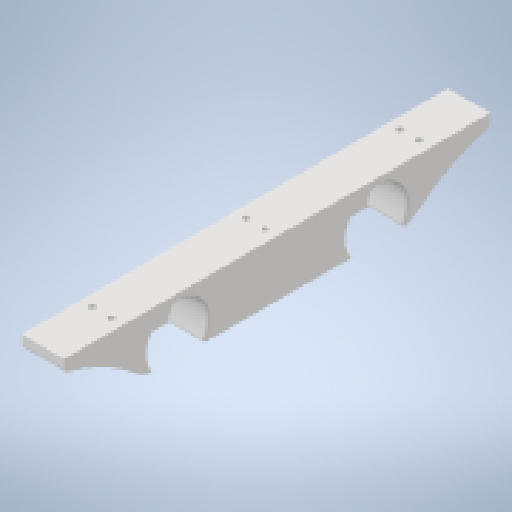
# Autodesk Inventor part: fasteners_motors
Saved by Autodesk Inventor 2023 (Build 270158000, 158)
## iProperties
Created: 2026-02-10
Part Number: fasteners_motors
Material: Типовые
Document SubType Name: Modeling
Designer: garin
Density: 1 g/cm^3
Appearance: По умолчанию
Author: garin
Autodesk Inventor part; units mm, degrees
ref_plane "YZ Plane" through (0, 0, 0) normal (1, 0, 0) x (0, 1, 0)
ref_plane "XY Plane" through (0, 0, 0) normal (0, 0, 1) x (1, 0, 0)
sketch "Эскиз1" plane through (0, 0, 0) normal (1, 0, 0) x (0, 1, 0)
  line L0 (0.0001, 0) -> (0.0001, -90)
  line L1 (0.0001, -90) -> (-4.9999, -90)
  line L2 (0.0001, -42) -> (0.0001, 0)
  circle A0 centre (-15.7559, -42) radius 12.6
  line L3 (-15.7559, -50.5) -> (-15.7559, -33.5) construction
  circle A1 centre (-15.7559, -50.5) radius 1.5
  circle A2 centre (-15.7559, -33.5) radius 1.5
  circle A3 centre (-15.7559, -42) radius 4
  line L4 (0.0001, 0) -> (-23.6599, 0)
  line L5 (-23.6599, 0) -> (-23.6599, -32.1874)
  line L6 (-23.6599, -32.1874) -> (-23.6599, -51.8126)
  arc A4 (-4.9999, -90) -> (-20.9999, -59) centre (-75.6064, -106.8131) ccw
  arc A5 (-23.6599, -51.8126) -> (-20.9999, -59) centre (-10.3066, -50.9566) ccw
  line L7 (40.5935, 0) -> (-48.1218, 0) construction
  line L8 (0.0001, 0) -> (0.0001, 90)
  line L9 (0.0001, 90) -> (-4.9999, 90)
  line L10 (0.0001, 42) -> (0.0001, 0)
  circle A6 centre (-15.7559, 42) radius 12.6
  line L11 (-15.7559, 50.5) -> (-15.7559, 33.5) construction
  circle A7 centre (-15.7559, 50.5) radius 1.5
  circle A8 centre (-15.7559, 33.5) radius 1.5
  circle A9 centre (-15.7559, 42) radius 4
  line L12 (-23.6599, 0) -> (-23.6599, 32.1874)
  line L13 (-23.6599, 32.1874) -> (-23.6599, 51.8126)
  arc A10 (-20.9999, 59) -> (-4.9999, 90) centre (-75.6064, 106.8131) ccw
  arc A11 (-20.9999, 59) -> (-23.6599, 51.8126) centre (-10.3066, 50.9566) ccw
  dimension "d34" = 90
  dimension "d35" = 5
  dimension "d38" = 25.2
  dimension "d39" = 8.5
  dimension "d40" = 17
  dimension "d41" = 3
  dimension "d42" = 3
  dimension "d43" = 8
  dimension "d44" = 23.66
  constraints: 28 end point, 14 symmetric about line, 12 centre point, 12 point on circle, 6 coincident, 3 perpendicular, 2 point on line, 1 horizontal, 1 vertical, 6 other
  measures "d34" distance of L0.start L0.end
  measures "d35" distance of L0.end L1.end
  measures "d38" diameter of A0
  measures "d39" distance of A0.centre L3.start
  measures "d40" distance of L3.start L3.end
  measures "d41" diameter of A1
  measures "d42" diameter of A2
  measures "d43" diameter of A3
  measures "d44" distance of L0.start L4.end
extrude "Выдавливание1" add sketch "Эскиз1" along normal blind 18 contours L0 L1 A4 A5 A0 L5 L4 | L4 L12 A6 A11 A10 L9 L8
extrude "Выдавливание2" add sketch "Эскиз1" along normal blind 3 contours A0 L6 | L13 A6 picked at (-22.3586, -42) picked at (-22.3586, 42)
chamfer "Фаска1" distance 2 angle 45 4 edges at (0, -17.2559, -33.5) (0, -17.2559, -50.5) (0, -17.2559, 50.5) (0, -17.2559, 33.5)
fillet "Сопряжение1" radius 1 6 edges at (10.5, -23.6599, -32.1874) (10.5, -23.6599, -51.8126) (18, -3.1559, -42) (18, -3.1559, 42) (10.5, -23.6599, 32.1874) (10.5, -23.6599, 51.8126)
fillet "Сопряжение2" radius 2 2 edges at (9, -4.9999, -90) (9, -4.9999, 90)
sketch "Эскиз2" plane through (0, 0.0001, 90) normal (0, 1, 0) x (1, 0, 0)
  line L0 (18, 180) -> (18, 0) projected
  line L1 (0, 0) -> (18, 0) projected
  line L2 (18, 180) -> (13, 180)
  line L3 (13, 180) -> (13, 0)
  line L4 (13, 0) -> (18, 0)
  line L5 (18, 0) -> (18, 180)
  line L6 (0, 180) -> (0, 0) projected
  line L7 (18, 0) -> (0, 0)
  line L8 (0, 0) -> (0, 25)
  line L9 (0, 25) -> (18, 25)
  line L10 (18, 25) -> (18, 0)
  line L11 (0, 180) -> (18, 180) projected
  line L12 (0, 0) -> (5, 0)
  line L13 (5, 0) -> (5, 180)
  line L14 (5, 180) -> (0, 180)
  line L15 (0, 180) -> (0, 0)
  line L16 (18, 180) -> (0, 180)
  line L17 (0, 180) -> (0, 155)
  line L18 (0, 155) -> (18, 155)
  line L19 (18, 155) -> (18, 180)
  line L20 (0, 90) -> (18, 90) construction
  circle A0 centre (13, 155) radius 1.35
  circle A1 centre (5, 155) radius 1.35
  circle A2 centre (13, 25) radius 1.35
  circle A3 centre (5, 25) radius 1.35
  circle A4 centre (13, 90) radius 1.35
  circle A5 centre (5, 90) radius 1.35
  circle A6 centre (13, 155) radius 2.1
  circle A7 centre (5, 155) radius 2.1
  circle A8 centre (5, 155) radius 3
  circle A9 centre (13, 155) radius 3
  circle A10 centre (13, 90) radius 2.1
  circle A11 centre (5, 90) radius 2.1
  circle A12 centre (5, 90) radius 3
  circle A13 centre (13, 90) radius 3
  circle A14 centre (13, 25) radius 2.1
  circle A15 centre (5, 25) radius 2.1
  circle A16 centre (5, 25) radius 3
  circle A17 centre (13, 25) radius 3
  dimension "d56" = 5
  dimension "d57" = 25
  dimension "d58" = 5
  dimension "d59" = 25
  dimension "d61" = 2.7
  dimension "d62" = 2.7
  dimension "d63" = 2.7
  dimension "d64" = 2.7
  dimension "d65" = 2.7
  dimension "d66" = 2.7
  dimension "d69" = 4.2
  dimension "d70" = 4.2
  dimension "d71" = 6
  dimension "d72" = 6
  dimension "d73" = 4.2
  dimension "d74" = 4.2
  dimension "d75" = 6
  dimension "d76" = 6
  constraints: 34 end point, 18 centre point, 14 point on line, 10 coincident, 8 parallel, 4 horizontal, 4 perpendicular, 4 symmetric about line, 3 midpoint, 4 other
  measures "d56" distance of L4.end L3.end
  measures "d57" distance of L7.end L8.end
  measures "d58" distance of L14.end L13.end
  measures "d59" distance of L17.end L16.end
  measures "d61" diameter of A0
  measures "d62" diameter of A1
  measures "d63" diameter of A2
  measures "d64" diameter of A3
  measures "d65" diameter of A4
  measures "d66" diameter of A5
  measures "d69" diameter of A6
  measures "d70" diameter of A7
  measures "d71" diameter of A8
  measures "d72" diameter of A9
  measures "d73" diameter of A10
  measures "d74" diameter of A11
  measures "d75" diameter of A12
  measures "d76" diameter of A13
ref_plane "РабПлоскость2" through (0, -10, 0) normal (0, 1, 0) x (-1, 0, 0)
ref_plane "РабПлоскость1" through (0, -5, 0) normal (0, 1, 0) x (-1, 0, 0)
extrude "Выдавливание3" cut sketch "Эскиз2" against normal blind 25 contours A0 L3 L18 | L18 L3 A0 | L3 L18 A0 | A2 L3 L9 | L9 L3 A2 | L3 A0 L18 | A1 L18 L13 | L13 L18 A1 | L9 A2 L3 | L3 A2 L9 | A4 L3 | L3 A4 | A1 L13 L18 | L13 A1 L18 | A3 L9 L13 | L13 L9 A3 | L9 L13 A3 | A5 L13 | L13 A5 | A3 L13 L9
extrude "Выдавливание4" cut sketch "Эскиз2" against normal blind 5 from surface at -5.0001 contours A6 L3 A0 L18 | L18 A0 L3 A6 | L3 A0 L18 A6 | A14 L3 A2 L9 | L9 A2 L3 A14 | A0 L3 L18 | L18 L3 A0 | A6 L18 A0 L3 | L3 L18 A0 | A7 L18 A1 L13 | L13 A1 L18 A7 | A2 L3 L9 | L9 L3 A2 | L3 A2 L9 A14 | A14 L9 A2 L3 | L3 A0 L18 | A10 L3 A4 | L3 A4 A10 | A7 L13 A1 L18 | A1 L18 L13 | L13 L18 A1 | L18 A1 L13 A7 | L9 A2 L3 | L3 A2 L9 | A4 L3 | L3 A4 | A1 L13 L18 | L13 A1 L18 | A15 L9 A3 L13 | L13 A3 L9 A15 | L9 A3 L13 A15 | A11 L13 A5 | L13 A5 A11 | A15 L13 A3 L9 | A3 L9 L13 | L13 L9 A3 | L9 L13 A3 | A5 L13 | L13 A5 | A3 L13 L9
extrude "Выдавливание5" cut sketch "Эскиз2" against normal blind 14 from surface at -10.0001 contours A9 L3 A6 L18 | L18 A6 L3 A9 | L3 A6 L18 A9 | A17 L3 A14 L9 | L9 A14 L3 A17 | A6 L3 A0 L18 | L18 A0 L3 A6 | A9 L18 A6 L3 | L3 A0 L18 A6 | A8 L18 A7 L13 | L13 A7 L18 A8 | A14 L3 A2 L9 | L9 A2 L3 A14 | L3 A14 L9 A17 | A17 L9 A14 L3 | A0 L3 L18 | L18 L3 A0 | A6 L18 A0 L3 | A13 L3 A10 | L3 A10 A13 | L3 L18 A0 | A8 L13 A7 L18 | A7 L18 A1 L13 | L13 A1 L18 A7 | L18 A7 L13 A8 | A2 L3 L9 | L9 L3 A2 | L3 A2 L9 A14 | A14 L9 A2 L3 | L3 A0 L18 | A10 L3 A4 | L3 A4 A10 | A7 L13 A1 L18 | A1 L18 L13 | L13 L18 A1 | L18 A1 L13 A7 | A16 L9 A15 L13 | L13 A15 L9 A16 | L9 A2 L3 | L3 A2 L9 | L9 A15 L13 A16 | A4 L3 | L3 A4 | A1 L13 L18 | A12 L13 A11 | L13 A11 A12 | A16 L13 A15 L9 | L13 A1 L18 | A15 L9 A3 L13 | L13 A3 L9 A15 | L9 A3 L13 A15 | A11 L13 A5 | L13 A5 A11 | A15 L13 A3 L9 | A3 L9 L13 | L13 L9 A3 | L9 L13 A3 | A5 L13 | L13 A5 | A3 L13 L9
